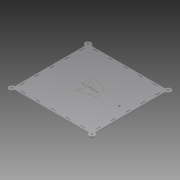
# Autodesk Inventor part: TopPlate
Saved by Autodesk Inventor 2015 SP1 (Build 190203100, 203)
## iProperties
Created: 2014-08-06
Part Number: TopPlate
Material: Acrylic, Clear
Document SubType Name: Modeling
Designer: Patrick Camilleri
Density: 1.19 g/cm^3
Appearance: Transparent - Clear
Mass: 654.149 g
Surface Area: 1962.87 cm^2
Volume: 549.705 cm^3
Author: Patrick Camilleri
Autodesk Inventor part; units mm, degrees
ref_plane "YZ Plane" through (0, 0, 0) normal (1, 0, 0) x (0, 1, 0)
ref_plane "XZ Plane" through (0, 0, 0) normal (0, 1, 0) x (-1, 0, 0)
ref_plane "XY Plane" through (0, 0, 0) normal (0, 0, 1) x (1, 0, 0)
sketch "Sketch1" plane through (0, 0, 0) normal (0, 0, 1) x (1, 0, 0)
  line L0 (-177, -128) -> (92, -128)
  line L1 (92, -128) -> (92, 128)
  line L2 (92, 128) -> (-177, 128)
  line L3 (-177, 128) -> (-177, -128)
  line L4 (-177, 0) -> (92, 0) construction
  line L5 (0, -128) -> (0, 128) construction
  point P0 (0, 0)
  point P1 (0, 0)
  dimension "d160" = 256
  dimension "d161" = 177
  dimension "d162" = 92
  constraints: 12 end point, 3 midpoint, 2 parallel, 2 perpendicular, 2 point on line, 1 coincident, 1 horizontal
  measures "d160" distance of L0.end L1.end
  measures "d161" distance between parallel lines of L3 L5
  measures "d162" distance between parallel lines of L1 L5
extrude "Extrusion1" add sketch "Sketch1" along normal blind 5
sketch "Sketch2" plane through (0, 0, 5) normal (0, 0, 1) x (1, 0, 0)
  line L0 (-171.925, 7.5) -> (-169.075, 7.5)
  line L1 (-169.075, 7.5) -> (-169.075, -7.5)
  line L2 (-169.075, -7.5) -> (-171.925, -7.5)
  line L3 (-171.925, -7.5) -> (-171.925, 7.5)
  line L4 (-171.925, 7.5) -> (-169.075, -7.5) construction
  line L5 (-169.075, 7.5) -> (-171.925, -7.5) construction
  line L6 (-177, -128) -> (92, -128) projected
  line L7 (92, -128) -> (92, 128) projected
  line L8 (92, 128) -> (-177, 128) projected
  line L9 (-177, 128) -> (-177, -128) projected
  line L10 (84.075, -7.5) -> (86.925, -7.5)
  line L11 (86.925, -7.5) -> (86.925, 7.5)
  line L12 (86.925, 7.5) -> (84.075, 7.5)
  line L13 (84.075, 7.5) -> (84.075, -7.5)
  line L14 (84.075, -7.5) -> (86.925, 7.5) construction
  line L15 (86.925, -7.5) -> (84.075, 7.5) construction
  line L16 (-170.5, -121.5) -> (85.5, -121.5) construction
  line L17 (85.5, -121.5) -> (85.5, 121.5) construction
  line L18 (85.5, 121.5) -> (-170.5, 121.5) construction
  line L19 (-170.5, 121.5) -> (-170.5, -121.5) construction
  point P0 (0, 0)
  point P1 (-170.5, 0)
  point P2 (85.5, 0)
  point P3 (85.5, 0)
  point P4 (-170.5, 0)
  dimension "d77" = 2.85
  dimension "d78" = 15
  dimension "d163" = 2.85
  dimension "d164" = 15
  dimension "d187" = 6.5
  constraints: 32 end point, 8 midpoint, 4 parallel, 2 horizontal, 2 perpendicular, 3 other
  measures "d77" distance of L1.end L2.end
  measures "d78" distance of L0.end L1.end
  measures "d163" distance of L12.end L11.end
  measures "d164" distance of L11.end L10.end
  measures "d187" distance between parallel lines of L9 L19
extrude "Extrusion3" cut sketch "Sketch2" against normal through all contours L0 L1 L2 L3 | L13 L12 L11 L10
sketch "Sketch3" plane through (0, 0, 5) normal (0, 0, 1) x (1, 0, 0)
  line L0 (-152.5, 122.925) -> (-137.5, 122.925)
  line L1 (-137.5, 122.925) -> (-137.5, 120.075)
  line L2 (-137.5, 120.075) -> (-152.5, 120.075)
  line L3 (-152.5, 120.075) -> (-152.5, 122.925)
  line L4 (-152.5, 122.925) -> (-137.5, 120.075) construction
  line L5 (-137.5, 122.925) -> (-152.5, 120.075) construction
  line L6 (-152.5, -120.075) -> (-137.5, -120.075)
  line L7 (-137.5, -120.075) -> (-137.5, -122.925)
  line L8 (-137.5, -122.925) -> (-152.5, -122.925)
  line L9 (-152.5, -122.925) -> (-152.5, -120.075)
  line L10 (-152.5, -120.075) -> (-137.5, -122.925) construction
  line L11 (-137.5, -120.075) -> (-152.5, -122.925) construction
  line L12 (-171.925, -7.5) -> (-171.925, 7.5) projected
  line L13 (-171.925, 7.5) -> (-169.075, 7.5) projected
  line L14 (-169.075, 7.5) -> (-169.075, -7.5) projected
  line L15 (-169.075, -7.5) -> (-171.925, -7.5) projected
  line L16 (-177, -128) -> (92, -128) projected
  line L17 (92, 128) -> (-177, 128) projected
  line L18 (-177, 128) -> (-177, -128) projected
  point P0 (0, 0)
  point P1 (-145, 121.5)
  point P2 (-145, -121.5)
  dimension "d125" = 15
  dimension "d126" = 2.85
  dimension "d128" = 15
  dimension "d129" = 2.85
  dimension "d198" = 32
  dimension "d199" = 6.5
  dimension "d200" = 32
  dimension "d201" = 6.5
  constraints: 24 end point, 4 midpoint, 4 parallel, 2 horizontal, 2 perpendicular
  measures "d125" distance of L1.end L2.end
  measures "d126" distance of L0.end L1.end
  measures "d128" distance of L7.end L8.end
  measures "d129" distance of L6.end L7.end
  measures "d198" distance from line of L18 point (-145, 121.5)
  measures "d199" distance from line of L17 point (-145, 121.5)
  measures "d200" distance from line of L18 point (-145, -121.5)
  measures "d201" distance from line of L16 point (-145, -121.5)
extrude "Extrusion4" cut sketch "Sketch3" against normal through all contours L0 L1 L2 L3 | L6 L7 L8 L9
pattern_linear "Rectangular Pattern1" count 5 spacing 50 along (1, 0, 0) of "Extrusion4"
pattern_linear "Rectangular Pattern2" count 3 spacing 50 along (0, -1, 0) of "Extrusion3"
pattern_linear "Rectangular Pattern3" count 3 spacing 50 along (0, 1, 0) of "Extrusion3"
sketch "Sketch7" plane through (0, 0, 5) normal (0, 0, 1) x (1, 0, 0)
  circle A0 centre (-177, -128) radius 10
  circle A1 centre (92, -128) radius 10
  point P0 (0, 0)
  dimension "d165" = 20
  dimension "d166" = 20
  constraints: 2 centre point, 2 coincident
  measures "d165" diameter of A0
  measures "d166" diameter of A1
extrude "Extrusion6" add sketch "Sketch7" against normal blind 6
mirror "Mirror7" about plane through (0, 0, 0) normal (0, 1, 0) of "Extrusion6"
hole "Hole6" at (-177, -128, 5) direction (0, 0, -1) diameter 6 end through all
hole "Hole7" at (92, -128, 5) direction (0, 0, -1) diameter 6 end through all
mirror "Mirror8" about plane through (0, 0, 0) normal (0, 1, 0) of "Hole6", "Hole7"
sketch "Sketch9" plane through (0, 0, 5) normal (0, 0, 1) x (1, 0, 0)
  line L0 (-169.075, 7.5) -> (-169.075, -7.5) projected
  line L1 (53.075, 3) -> (59.075, 3)
  line L2 (59.075, 3) -> (59.075, -3)
  line L3 (59.075, -3) -> (53.075, -3)
  line L4 (53.075, -3) -> (53.075, 3)
  point P0 (0, 0)
  point P1 (53.075, 0)
  point P2 (53.075, 0)
  dimension "d193" = 222.15
  dimension "d194" = 6
  dimension "d195" = 6
  constraints: 8 end point, 2 parallel, 1 coincident, 1 horizontal, 1 midpoint, 1 perpendicular
  measures "d193" distance from line of point (53.075, 0) L0
  measures "d194" distance of L2.end L3.end
  measures "d195" distance of L1.end L2.end
extrude "SquareHole" cut sketch "Sketch9" against normal through all
sketch "SpiNNaker" plane through (0, 0, 5) normal (0, 0, 1) x (1, 0, 0)
  line L0 (-75.2008, 7.9321) -> (-4.322, 7.9321) construction
  line L1 (-4.322, 7.9321) -> (-4.322, -5.5231) construction
  line L2 (-4.322, -5.5231) -> (-75.2008, -5.5231) construction
  line L3 (-75.2008, -5.5231) -> (-75.2008, 7.9321) construction
  line L4 (-74.8349, 2.1853) -> (-73.4203, 2.3378)
  spline S0 degree 2 poles (-73.4203, 2.3378) (-73.2923, 1.5451) (-72.5118, 0.8012) (-71.8532, 0.8012) knots 0 0 0 1 2 2 2
  spline S1 degree 2 poles (-71.8532, 0.8012) (-71.152, 0.8012) (-70.4386, 1.4597) (-70.4386, 1.9049) knots 0 0 0 1 2 2 2
  spline S2 degree 2 poles (-70.4386, 1.9049) (-70.4386, 2.1914) (-70.7374, 2.5878) (-71.1093, 2.7341) knots 0 0 0 1 2 2 2
  spline S3 degree 2 poles (-71.1093, 2.7341) (-71.3654, 2.8317) (-72.274, 3.0817) knots 0 0 0 1 1 1
  spline S4 degree 2 poles (-72.274, 3.0817) (-73.4386, 3.4049) (-73.9081, 3.8744) knots 0 0 0 1 1 1
  spline S5 degree 2 poles (-73.9081, 3.8744) (-74.5727, 4.5329) (-74.5727, 5.478) knots 0 0 0 1 1 1
  spline S6 degree 2 poles (-74.5727, 5.478) (-74.5727, 6.0939) (-73.9508, 7.1549) (-72.7801, 7.7097) (-71.9508, 7.7097) knots 0 0 0 1 2 3 3 3
  spline S7 degree 2 poles (-71.9508, 7.7097) (-70.5971, 7.7097) (-69.2313, 6.3927) (-69.1947, 5.289) knots 0 0 0 1 2 2 2
  line L5 (-69.1947, 5.289) -> (-70.6459, 5.2158)
  spline S8 degree 2 poles (-70.6459, 5.2158) (-70.7374, 5.8317) (-71.3532, 6.3744) (-71.963, 6.3744) knots 0 0 0 1 2 2 2
  spline S9 degree 2 poles (-71.963, 6.3744) (-72.5971, 6.3744) (-72.9508, 6.0878) knots 0 0 0 1 1 1
  spline S10 degree 2 poles (-72.9508, 6.0878) (-73.1825, 5.8988) (-73.1825, 5.5878) knots 0 0 0 1 1 1
  spline S11 degree 2 poles (-73.1825, 5.5878) (-73.1825, 5.3073) (-72.9691, 5.1) knots 0 0 0 1 1 1
  spline S12 degree 2 poles (-72.9691, 5.1) (-72.6947, 4.8439) (-70.5727, 4.289) (-69.5605, 3.6975) (-68.9874, 2.667) (-68.9874, 1.9049) knots 0 0 0 1 2 3 4 4 4
  spline S13 degree 2 poles (-68.9874, 1.9049) (-68.9874, 1.2219) (-69.6764, 0.0207) (-70.9325, -0.5647) (-71.8654, -0.5647) knots 0 0 0 1 2 3 3 3
  spline S14 degree 2 poles (-71.8654, -0.5647) (-73.2313, -0.5647) (-74.6947, 0.8378) (-74.8349, 2.1853) knots 0 0 0 1 2 2 2
  line L6 (-67.8105, 5.3744) -> (-66.524, 5.3744)
  line L7 (-66.524, 5.3744) -> (-66.524, 4.5207)
  spline S15 degree 2 poles (-66.524, 4.5207) (-66.274, 4.9597) (-65.4203, 5.5024) (-64.902, 5.5024) knots 0 0 0 1 2 2 2
  spline S16 degree 2 poles (-64.902, 5.5024) (-63.9935, 5.5024) (-62.7252, 3.9231) (-62.7252, 2.5085) knots 0 0 0 1 2 2 2
  spline S17 degree 2 poles (-62.7252, 2.5085) (-62.7252, 1.0573) (-63.9996, -0.5525) (-64.9081, -0.5525) knots 0 0 0 1 2 2 2
  spline S18 degree 2 poles (-64.9081, -0.5525) (-65.341, -0.5525) (-66.0423, -0.1683) (-66.4325, 0.2951) knots 0 0 0 1 2 2 2
  line L8 (-66.4325, 0.2951) -> (-66.4325, -2.6317)
  line L9 (-66.4325, -2.6317) -> (-67.8105, -2.6317)
  line L10 (-67.8105, -2.6317) -> (-67.8105, 5.3744)
  spline S19 degree 2 poles (-66.4508, 2.5756) (-66.4508, 1.6) (-65.7496, 0.667) (-65.2496, 0.667) knots 0 0 0 1 2 2 2
  spline S20 degree 2 poles (-65.2496, 0.667) (-64.7679, 0.667) (-64.1276, 1.5207) (-64.1276, 2.4963) knots 0 0 0 1 2 2 2
  spline S21 degree 2 poles (-64.1276, 2.4963) (-64.1276, 3.4049) (-64.7862, 4.289) (-65.274, 4.289) knots 0 0 0 1 2 2 2
  spline S22 degree 2 poles (-65.274, 4.289) (-65.7801, 4.289) (-66.4508, 3.4231) (-66.4508, 2.5756) knots 0 0 0 1 2 2 2
  line L11 (-61.6337, -0.4244) -> (-61.6337, 5.3744)
  line L12 (-61.6337, 5.3744) -> (-60.2557, 5.3744)
  line L13 (-60.2557, 5.3744) -> (-60.2557, -0.4244)
  line L14 (-60.2557, -0.4244) -> (-61.6337, -0.4244)
  line L15 (-61.6337, 6.1549) -> (-61.6337, 7.5756)
  line L16 (-61.6337, 7.5756) -> (-60.2557, 7.5756)
  line L17 (-60.2557, 7.5756) -> (-60.2557, 6.1549)
  line L18 (-60.2557, 6.1549) -> (-61.6337, 6.1549)
  line L19 (-46.8539, -0.4244) -> (-48.5913, -0.4244)
  line L20 (-48.5913, -0.4244) -> (-51.3661, 5.1509)
  line L21 (-51.3661, 5.1509) -> (-51.3661, -0.4244)
  line L22 (-51.3661, -0.4244) -> (-53.0192, -0.4244)
  line L23 (-53.0192, -0.4244) -> (-53.0192, 7.5756)
  line L24 (-53.0192, 7.5756) -> (-50.802, 7.5756)
  line L25 (-50.802, 7.5756) -> (-48.5071, 2.9921)
  line L26 (-48.5071, 2.9921) -> (-48.5071, 7.5756)
  line L27 (-48.5071, 7.5756) -> (-46.8539, 7.5756)
  line L28 (-46.8539, 7.5756) -> (-46.8539, -0.4244)
  line L29 (-39.2299, -0.4244) -> (-40.9673, -0.4244)
  line L30 (-40.9673, -0.4244) -> (-43.7421, 5.1509)
  line L31 (-43.7421, 5.1509) -> (-43.7421, -0.4244)
  line L32 (-43.7421, -0.4244) -> (-45.3952, -0.4244)
  line L33 (-45.3952, -0.4244) -> (-45.3952, 7.5756)
  line L34 (-45.3952, 7.5756) -> (-43.178, 7.5756)
  line L35 (-43.178, 7.5756) -> (-40.8831, 2.9921)
  line L36 (-40.8831, 2.9921) -> (-40.8831, 7.5756)
  line L37 (-40.8831, 7.5756) -> (-39.2299, 7.5756)
  line L38 (-39.2299, 7.5756) -> (-39.2299, -0.4244)
  spline S23 degree 2 poles (-34.8733, 0.2174) (-35.0484, 0.0553) (-35.3207, -0.204) (-35.5541, -0.3337) knots 0 0 0 1 2 2 2
  spline S24 degree 2 poles (-35.5541, -0.3337) (-35.781, -0.4568) (-36.2153, -0.5865) (-36.6043, -0.5865) knots 0 0 0 1 2 2 2
  spline S25 degree 2 poles (-36.6043, -0.5865) (-37.3239, -0.5865) (-38.2769, 0.4897) (-38.2769, 1.3065) knots 0 0 0 1 2 2 2
  spline S26 degree 2 poles (-38.2769, 1.3065) (-38.2769, 1.9743) (-37.7907, 2.8041) (-37.3369, 3.044) knots 0 0 0 1 2 2 2
  spline S27 degree 2 poles (-37.3369, 3.044) (-36.8766, 3.2903) (-35.5994, 3.4848) (-34.8669, 3.5367) knots 0 0 0 1 2 2 2
  line L39 (-34.8669, 3.5367) -> (-34.8669, 3.5691)
  spline S28 degree 2 poles (-34.8669, 3.5691) (-34.8669, 4.0683) (-35.5281, 4.4508) (-36.1894, 4.4508) knots 0 0 0 1 2 2 2
  spline S29 degree 2 poles (-36.1894, 4.4508) (-36.4941, 4.4508) (-37.298, 4.2109) (-37.6805, 4.0229) knots 0 0 0 1 2 2 2
  line L40 (-37.6805, 4.0229) -> (-37.8231, 4.0229)
  line L41 (-37.8231, 4.0229) -> (-37.8231, 5.4816)
  spline S30 degree 2 poles (-37.8231, 5.4816) (-37.5703, 5.5594) (-36.4487, 5.7798) (-35.8782, 5.7798) knots 0 0 0 1 2 2 2
  spline S31 degree 2 poles (-35.8782, 5.7798) (-34.4779, 5.7798) (-33.1943, 4.7425) (-33.1943, 3.6793) knots 0 0 0 1 2 2 2
  line L42 (-33.1943, 3.6793) -> (-33.1943, -0.4244)
  line L43 (-33.1943, -0.4244) -> (-34.8733, -0.4244)
  line L44 (-34.8733, -0.4244) -> (-34.8733, 0.2174)
  line L45 (-34.8733, 1.1509) -> (-34.8733, 2.4022)
  spline S32 degree 2 poles (-34.8733, 2.4022) (-35.3077, 2.3568) (-35.8393, 2.2855) (-36.0921, 2.1817) knots 0 0 0 1 2 2 2
  spline S33 degree 2 poles (-36.0921, 2.1817) (-36.3191, 2.0975) (-36.5654, 1.7474) (-36.5654, 1.4621) knots 0 0 0 1 2 2 2
  spline S34 degree 2 poles (-36.5654, 1.4621) (-36.5654, 1.0407) (-36.1505, 0.7231) (-35.7485, 0.7231) knots 0 0 0 1 2 2 2
  spline S35 degree 2 poles (-35.7485, 0.7231) (-35.5281, 0.7231) (-35.0614, 0.95) (-34.8733, 1.1509) knots 0 0 0 1 2 2 2
  line L46 (-26.5168, -0.4244) -> (-28.5265, -0.4244)
  line L47 (-28.5265, -0.4244) -> (-29.9917, 2.2012)
  line L48 (-29.9917, 2.2012) -> (-30.251, 1.8122)
  line L49 (-30.251, 1.8122) -> (-30.251, -0.4244)
  line L50 (-30.251, -0.4244) -> (-31.943, -0.4244)
  line L51 (-31.943, -0.4244) -> (-31.943, 7.9321)
  line L52 (-31.943, 7.9321) -> (-30.251, 7.9321)
  line L53 (-30.251, 7.9321) -> (-30.251, 3.2579)
  line L54 (-30.251, 3.2579) -> (-28.6562, 5.6112)
  line L55 (-28.6562, 5.6112) -> (-26.6594, 5.6112)
  line L56 (-26.6594, 5.6112) -> (-28.5524, 3.0116)
  line L57 (-28.5524, 3.0116) -> (-26.5168, -0.4244)
  spline S36 degree 2 poles (-23.204, -0.5865) (-24.734, -0.5865) (-26.3742, 1.0472) (-26.3742, 2.5578) knots 0 0 0 1 2 2 2
  spline S37 degree 2 poles (-26.3742, 2.5578) (-26.3742, 4.0359) (-24.8507, 5.7992) (-23.4763, 5.7992) knots 0 0 0 1 2 2 2
  spline S38 degree 2 poles (-23.4763, 5.7992) (-22.2315, 5.7992) (-20.9738, 4.3017) (-20.9738, 2.9143) knots 0 0 0 1 2 2 2
  line L58 (-20.9738, 2.9143) -> (-20.9738, 2.2336)
  line L59 (-20.9738, 2.2336) -> (-24.6821, 2.2336)
  spline S39 degree 2 poles (-24.6821, 2.2336) (-24.6562, 1.8122) (-24.3904, 1.2547) (-24.1635, 1.0861) knots 0 0 0 1 2 2 2
  spline S40 degree 2 poles (-24.1635, 1.0861) (-23.9495, 0.9176) (-23.3661, 0.7749) (-23.0225, 0.7749) knots 0 0 0 1 2 2 2
  spline S41 degree 2 poles (-23.0225, 0.7749) (-22.7307, 0.7749) (-22.1602, 0.9176) (-21.9203, 1.0407) knots 0 0 0 1 2 2 2
  spline S42 degree 2 poles (-21.9203, 1.0407) (-21.7129, 1.138) (-21.3628, 1.3779) (-21.2526, 1.4686) knots 0 0 0 1 2 2 2
  line L60 (-21.2526, 1.4686) -> (-21.0711, 1.4686)
  line L61 (-21.0711, 1.4686) -> (-21.0711, -0.0873)
  spline S43 degree 2 poles (-21.0711, -0.0873) (-21.2785, -0.1781) (-21.6221, -0.3337) (-21.9203, -0.4115) knots 0 0 0 1 2 2 2
  spline S44 degree 2 poles (-21.9203, -0.4115) (-22.1991, -0.4957) (-22.7826, -0.5865) (-23.204, -0.5865) knots 0 0 0 1 2 2 2
  spline S45 degree 2 poles (-22.64, 3.3681) (-22.6529, 3.9646) (-23.1262, 4.5934) (-23.6059, 4.5934) knots 0 0 0 1 2 2 2
  spline S46 degree 2 poles (-23.6059, 4.5934) (-24.0986, 4.5934) (-24.6562, 3.9321) (-24.6886, 3.3681) knots 0 0 0 1 2 2 2
  line L62 (-24.6886, 3.3681) -> (-22.64, 3.3681)
  line L63 (-16.4617, 3.8284) -> (-16.6043, 3.8284)
  spline S47 degree 2 poles (-16.6043, 3.8284) (-16.6951, 3.8673) (-17.0646, 3.9062) (-17.285, 3.9062) knots 0 0 0 1 2 2 2
  spline S48 degree 2 poles (-17.285, 3.9062) (-17.5508, 3.9062) (-18.1408, 3.7312) (-18.4131, 3.6145) knots 0 0 0 1 2 2 2
  line L64 (-18.4131, 3.6145) -> (-18.4131, -0.4244)
  line L65 (-18.4131, -0.4244) -> (-20.1051, -0.4244)
  line L66 (-20.1051, -0.4244) -> (-20.1051, 5.6112)
  line L67 (-20.1051, 5.6112) -> (-18.4131, 5.6112)
  line L68 (-18.4131, 5.6112) -> (-18.4131, 4.7425)
  spline S49 degree 2 poles (-18.4131, 4.7425) (-18.2964, 4.8592) (-17.8879, 5.2223) (-17.7194, 5.3325) knots 0 0 0 1 2 2 2
  spline S50 degree 2 poles (-17.7194, 5.3325) (-17.5314, 5.4556) (-17.0451, 5.6307) (-16.8312, 5.6307) knots 0 0 0 1 2 2 2
  spline S51 degree 2 poles (-16.8312, 5.6307) (-16.7469, 5.6307) (-16.546, 5.6177) (-16.4617, 5.6112) knots 0 0 0 1 2 2 2
  line L69 (-16.4617, 5.6112) -> (-16.4617, 3.8284)
  point P0 (0, 0)
  constraints: 2 other
sketch "Sail" plane through (0, 0, 5) normal (0, 0, 1) x (1, 0, 0)
  spline S0 degree 4 poles (-74.7671, 35.7975) (-44.8987, 38.4161) (-13.3799, 29.1988) (6.0878, -10.0846) (-16.7434, -17.9627) (-29.2684, -22.2846) knots 0 0 0 0 0 0.533696 1 1 1 1 1
  spline S1 degree 2 poles (-74.7671, 35.7975) (-44.8987, 3.913) (-62.4454, -31.0567) knots 0 0 0 1 1 1
  spline S2 degree 1 poles (-62.4454, -31.0567) (-28.4498, -14.9812) knots 0 0 1 1
  line L0 (-28.4498, -14.9812) -> (-29.2684, -22.2846)
  line L1 (-74.7671, 35.7975) -> (-44.8987, 38.4161) construction
  line L2 (-44.8987, 38.4161) -> (-13.3799, 29.1988) construction
  line L3 (-13.3799, 29.1988) -> (6.0878, -10.0846) construction
  line L4 (6.0878, -10.0846) -> (-16.7434, -17.9627) construction
  line L5 (-16.7434, -17.9627) -> (-29.2684, -22.2846) construction
  line L6 (-74.7671, 35.7975) -> (-44.8987, 3.913) construction
  line L7 (-44.8987, 3.913) -> (-62.4454, -31.0567) construction
  line L8 (-62.4454, -31.0567) -> (-28.4498, -14.9812) construction
  spline S3 degree 2 poles (-72.6358, 35.0781) (-44.8987, 3.913) (-60.4918, -29.101) knots 0 0 0 1 1 1
  spline S4 degree 1 poles (-60.4918, -29.101) (-28.253, -13.8562) knots 0 0 1 1
  spline S5 degree 4 poles (-72.6358, 35.0781) (-45.8382, 37.1068) (-18.7423, 29.3933) (1.5139, -3.3748) (-12.0268, -13.5718) (-18.1796, -16.545) knots 0 0 0 0 0 1 2 2 2 2 2
  line L9 (-72.6358, 35.0781) -> (-45.8382, 37.1068) construction
  line L10 (-45.8382, 37.1068) -> (-18.7423, 29.3933) construction
  line L11 (-12.0268, -13.5718) -> (-18.1796, -16.545) construction
  line L12 (-72.6358, 35.0781) -> (-44.8987, 3.913) construction
  line L13 (-44.8987, 3.913) -> (-60.4918, -29.101) construction
  line L14 (-60.4918, -29.101) -> (-28.253, -13.8562) construction
  line L15 (-18.7423, 29.3933) -> (1.5139, -3.3748) construction
  line L16 (1.5139, -3.3748) -> (-12.0268, -13.5718) construction
  line L17 (-18.1796, -16.545) -> (-19.0711, -11.2168) construction
  line L18 (-19.0711, -11.2168) -> (-28.253, -13.8562) construction
  spline S6 degree 2 poles (-18.1796, -16.545) (-19.0711, -11.2168) (-28.253, -13.8562) knots 1 1 1 2 2 2
  line L19 (-27.5653, -14.405) -> (-28.2904, -20.9134)
  line L20 (-27.5653, -14.405) -> (-19.7983, -12.2945) construction
  line L21 (-19.7983, -12.2945) -> (-19.1423, -17.1296) construction
  spline S7 degree 2 poles (-27.5653, -14.405) (-19.7983, -12.2945) (-19.1423, -17.1296) knots 1 1 1 2 2 2
  line L22 (-28.2904, -20.9134) -> (-23.0059, -19.4574) construction
  line L23 (-23.0059, -19.4574) -> (-19.1423, -17.1296) construction
  spline S8 degree 2 poles (-28.2904, -20.9134) (-23.0059, -19.4574) (-19.1423, -17.1296) knots 1 1 1 2 2 2
  point P0 (0, 0)
  constraints: 4 end point, 1 coincident, 1 parallel, 27 other
emboss "SpiNNaker_Emboss" sketch "SpiNNaker" operation cut depth 1 direction (0, 0, -1)
emboss "Sail_Emboss" sketch "Sail" operation cut depth 1 direction (0, 0, -1)
equation "\"d166\" = d165"
equation "\"kerf\" = 0.15"
body "Solid1"
